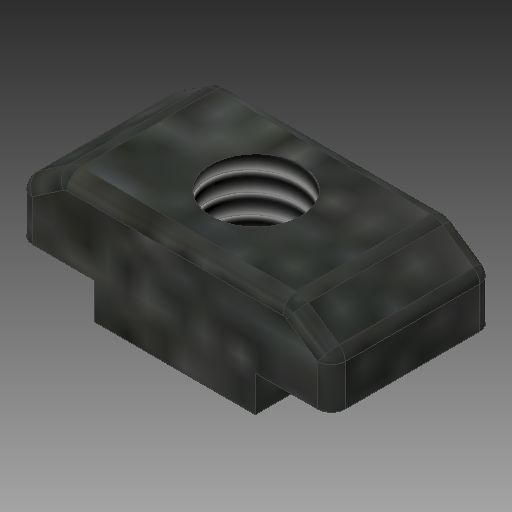
# Autodesk Inventor part: Noix M4
Saved by Autodesk Inventor 2017 (Build 210142000, 142)
## iProperties
Company: FABLAB Frenchmakers
Part Number: Noix M4
Material: Acier
Document SubType Name: Modeling
Designer: FABLAB Frenchmakers
Density: 7.85 g/cm^3
Appearance: Plaque
Mass: 1.44595 g
Surface Area: 2.64494 cm^2
Volume: 0.184197 cm^3
Stock Number: 1420-01-12
Project: 1420 Vauban 3D XL
Autodesk Inventor part; units mm, degrees
ref_plane "YZ Plane" through (0, 0, 0) normal (1, 0, 0) x (0, 1, 0)
ref_plane "XZ Plane" through (0, 0, 0) normal (0, 1, 0) x (-1, 0, 0)
ref_plane "XY Plane" through (0, 0, 0) normal (0, 0, 1) x (1, 0, 0)
sketch "Esquisse1" plane through (0, 0, 0) normal (0, 0, 1) x (1, 0, 0)
  line L0 (-5.65, 0) -> (5.65, 0)
  line L1 (5.65, 0) -> (5.65, 1.75)
  line L2 (5.65, 1.75) -> (4.125, 2.8)
  line L3 (4.125, 2.8) -> (-4.125, 2.8)
  line L4 (-4.125, 2.8) -> (-5.65, 1.75)
  line L5 (-5.65, 1.75) -> (-5.65, 0)
  point P0 (0, 0)
  dimension "d0" = 11.3
  dimension "d1" = 2.8
  dimension "d2" = 8.25
  dimension "d3" = 5.65
  dimension "d4" = 1.75
  constraints: 12 end point, 2 horizontal alignment, 2 parallel, 1 equal length, 1 horizontal, 1 perpendicular
  measures "d0" distance between parallel lines of L1 L5
  measures "d1" distance between parallel lines of L0 L3
  measures "d2" distance of L2.end L3.end
  measures "d3" distance from line of point (0, 0) L1
  measures "d4" distance of L4.end L0.start
extrude "Extrusion1" add sketch "Esquisse1" along normal mid plane 5.85
sketch "Esquisse2" plane through (-5.65, 0, 2.925) normal (0, -1, 0) x (1, 0, 0)
  line L0 (2.75, -5.85) -> (8.55, -5.85)
  line L1 (8.55, -5.85) -> (8.55, 0)
  line L2 (8.55, 0) -> (2.75, 0)
  line L3 (2.75, 0) -> (2.75, -5.85)
  line L4 (2.75, -5.85) -> (8.55, 0) construction
  line L5 (8.55, -5.85) -> (2.75, 0) construction
  line L6 (0, 0) -> (11.3, 0) projected
  point P0 (5.65, -2.925)
  dimension "d7" = 5.8
  constraints: 12 end point, 2 midpoint, 2 parallel, 1 collinear, 1 horizontal, 1 perpendicular
  measures "d7" distance between parallel lines of L1 L3
extrude "Extrusion2" add sketch "Esquisse2" along normal blind 1.3
sketch "Esquisse3" plane through (-4.125, 2.8, 2.925) normal (0, 1, 0) x (1, 0, 0)
  point P0 (4.125, 2.925)
  point P1 (4.125, 2.925)
  constraints: 1 coincident
hole "Perçage1" at (0, 2.8, 0) direction (0, -1, 0) diameter 3.242 depth 11.8 tip angle 118 thread size "M4x0.7" class "6H" standard "ISO Metric profile"
fillet "Congé1" radius 0.5 2 edges at (-5.65, 1.75, 0) (5.65, 1.75, 0)
fillet "Congé2" radius 0.75 2 edges at (4.125, 2.8, 0) (-4.125, 2.8, 0)
fillet "Congé3" radius 0.5 18 edges at (-5.5926, 1.7198, 2.925) (-5.65, 0.7436, 2.925) (-4.1145, 2.7662, 2.925) (0, 2.8, 2.925) (4.1145, 2.7662, 2.925) (4.8753, 2.2834, 2.925) (5.5926, 1.7198, 2.925) (5.65, 0.7436, 2.925) (-4.8753, 2.2834, 2.925) (-4.1145, 2.7662, -2.925) (0, 2.8, -2.925) (4.1145, 2.7662, -2.925) (4.8753, 2.2834, -2.925) (5.5926, 1.7198, -2.925) (5.65, 0.7436, -2.925) (-5.5926, 1.7198, -2.925) (-5.65, 0.7436, -2.925) (-4.8753, 2.2834, -2.925)
equation "\"d3\" = 0.5 * d0"
